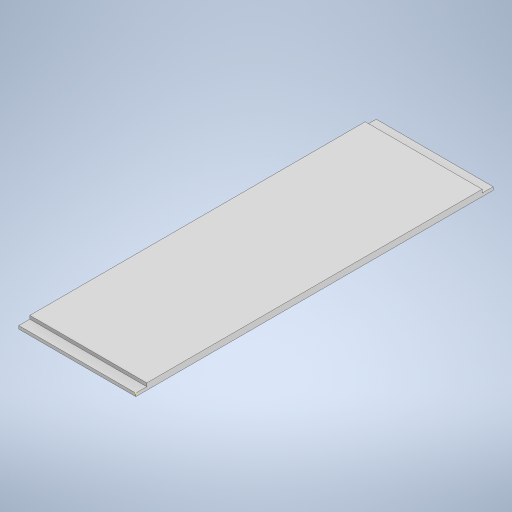
# Autodesk Inventor part: Part2
Saved by Autodesk Inventor 2024 (Build 280153000, 153)
## iProperties
Created: 2025-02-26
Part Number: Part2
Material: Generic
Document SubType Name: Modeling
Designer: vandevelde.wout
Density: 1 g/cm^3
Appearance: Default
Author: vandevelde.wout
Autodesk Inventor part; units mm, degrees
ref_plane "YZ Plane" through (0, 0, 0) normal (1, 0, 0) x (0, 1, 0)
ref_plane "XZ Plane" through (0, 0, 0) normal (0, 1, 0) x (-1, 0, 0)
ref_plane "XY Plane" through (0, 0, 0) normal (0, 0, 1) x (1, 0, 0)
sketch "Sketch1" plane through (0, 0, 0) normal (0, 1, 0) x (-1, 0, 0)
  line L0 (0, 0) -> (53, 0)
  line L1 (53, 0) -> (53, -162)
  line L2 (53, -162) -> (0, -162)
  line L3 (0, -162) -> (0, 0)
  dimension "d0" = 53
  dimension "d1" = 162
  constraints: 8 end point, 2 parallel, 1 horizontal, 1 perpendicular
  measures "d0" distance of L1.end L2.end
  measures "d1" distance of L0.end L1.end
extrude "Extrusion1" add sketch "Sketch1" along normal blind 1.4
sketch "Sketch2" plane through (0, 1.4, 0) normal (0, 1, 0) x (1, 0, 0)
  point P0 (0, 0)
sketch "Sketch3" plane through (0, 0, 0) normal (1, 0, 0) x (0, 0, -1)
  line L0 (162, 1.4) -> (0, 1.4) projected
  line L1 (5, 1.4) -> (5, 2.9)
  line L2 (5, 2.9) -> (157, 2.9)
  line L3 (157, 2.9) -> (157, 1.4)
  line L4 (0, 0) -> (0, 1.4) projected
  line L5 (162, 0) -> (162, 1.4) projected
  dimension "d4" = 5
  dimension "d5" = 1.5
  dimension "d6" = 5
  constraints: 6 end point, 2 perpendicular, 2 point on line, 1 vertical
  measures "d4" distance between parallel lines of L1 L4
  measures "d5" distance between parallel lines of L0 L2
  measures "d6" distance between parallel lines of L3 L5
extrude "Extrusion2" add sketch "Sketch3" against normal blind 53
body "Solid1"
